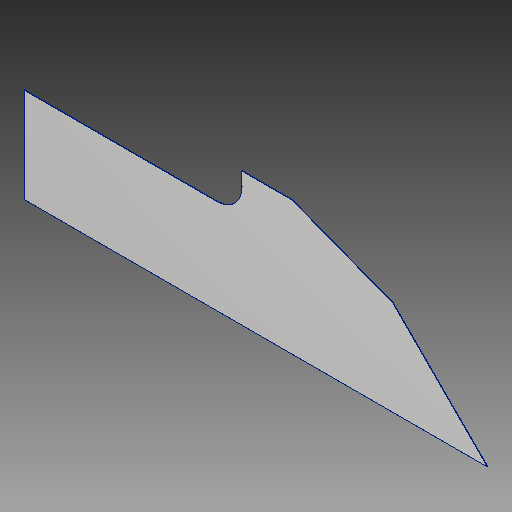
# Autodesk Inventor part: Side Plates
Saved by Autodesk Inventor 2019.4 (Build 234330000, 330)
## iProperties
Created: 2020-01-19
Part Number: Side Plates
Material: Aluminum 6061
Document SubType Name: Modeling
Designer: Mark
Mass: 472.2 g
Surface Area: 3519.77 cm^2
Volume: 174.889 cm^3
Density: 2.7 g/cm^3
Appearance: Aluminum - Flat
Author: Mark
Autodesk Inventor part; units mm, degrees
ref_plane "YZ Plane" through (0, 0, 0) normal (1, 0, 0) x (0, 1, 0)
ref_plane "XZ Plane" through (0, 0, 0) normal (0, 1, 0) x (-1, 0, 0)
ref_plane "XY Plane" through (0, 0, 0) normal (0, 0, 1) x (1, 0, 0)
sketch "Sketch1" plane through (0, 0, 0) normal (0, 0, 1) x (1, 0, 0)
  line L0 (-740, 0) -> (0, 0)
  line L1 (0, 0) -> (0, 190)
  line L2 (0, 190) -> (-740, 190)
  line L3 (-740, 190) -> (-740, 170)
  line L4 (0, -25.9599) -> (0, 190) construction
  line L5 (0, 0) -> (-740, 190) construction
  line L6 (0, 190) -> (190, 0)
  line L7 (190, 0) -> (0, 0)
  line L8 (-740, 190) -> (-740, 170)
  line L9 (-740, 190) -> (-720, 190) construction
  line L10 (-740, 170) -> (-740, 0)
  line L11 (0, 190) -> (-202.623, 268)
  line L12 (-202.623, 268) -> (-202.623, 190)
  line L13 (-202.623, 268) -> (-302.623, 268)
  line L14 (-302.623, 268) -> (-302.623, 190)
  line L15 (-302.623, 190) -> (-202.623, 190)
  line L16 (-202.623, 190) -> (-202.623, 268)
  dimension "d0" = 740
  dimension "d1" = 190
  dimension "d2" = 45
  dimension "d3" = 20
  dimension "d4" = 90
  dimension "d5" = 90
  dimension "d8" = 90
  dimension "d9" = 78
  dimension "d10" = 202.623
  dimension "d11" = 100
  constraints: 35 end point, 4 parallel, 4 perpendicular, 3 horizontal, 3 point on line, 1 collinear
  measures "d0" distance of L2.end L1.end
  measures "d1" distance of L0.end L1.end
  measures "d2" angle of L1 L6
  measures "d3" distance of L3.end L2.end
  measures "d4" angle of L8 L9
  measures "d5" angle of L0 L10
  measures "d8" angle of L2 L12
  measures "d9" distance of L11.end L12.end
  measures "d10" distance from line of L1.end L12
  measures "d11" distance of L15.end L14.end
extrude "Extrusion1" add sketch "Sketch1" along normal blind 1
fillet "Fillet1" radius 50 1 edges at (-302.623, 190, 0.5)
body "Solid1"
